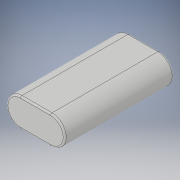
# Autodesk Inventor part: 4400mAh-LiIon-Battery
Saved by Autodesk Inventor 2019 (Build 230136000, 136)
## iProperties
Created: 2019-04-11
Part Number: 4400mAh-LiIon-Battery
Material: Generic
Document SubType Name: Modeling
Designer: Epsilon
Density: 1 g/cm^3
Appearance: Default
Author: Epsilon
Autodesk Inventor part; units mm, degrees
ref_plane "YZ Plane" through (0, 0, 0) normal (1, 0, 0) x (0, 1, 0)
ref_plane "XZ Plane" through (0, 0, 0) normal (0, 1, 0) x (-1, 0, 0)
ref_plane "XY Plane" through (0, 0, 0) normal (0, 0, 1) x (1, 0, 0)
sketch "Sketch1" plane through (0, 0, 0) normal (0, 1, 0) x (-1, 0, 0)
  line L0 (0, 0) -> (37, 0)
  line L1 (37, 0) -> (37, -69)
  line L2 (37, -69) -> (0, -69)
  line L3 (0, -69) -> (0, 0)
  dimension "d0" = 37
  dimension "d1" = 69
  constraints: 8 end point, 2 parallel, 1 horizontal, 1 perpendicular
  measures "d0" distance of L1.end L2.end
  measures "d1" distance of L0.end L1.end
extrude "Extrusion1" add sketch "Sketch1" along normal blind 18
fillet "Fillet1" radius 9 4 edges at (0, 18, -34.5) (0, 0, -34.5) (-37, 18, -34.5) (-37, 0, -34.5)
fillet "Fillet2" radius 1 16 edges at (0, 9, 0) (-2.636, 2.636, 0) (-2.636, 15.364, 0) (-18.5, 0, 0) (-34.364, 2.636, 0) (-34.364, 15.364, 0) (-37, 9, 0) (-18.5, 18, 0) (-34.364, 2.636, -69) (-34.364, 15.364, -69) (-37, 9, -69) (-18.5, 0, -69) (0, 9, -69) (-2.636, 2.636, -69) (-2.636, 15.364, -69) (-18.5, 18, -69)
body "Solid1"
